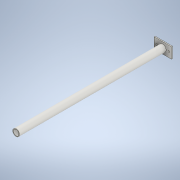
# Autodesk Inventor part: tubo_principal
Saved by Autodesk Inventor 2021 (Build 250183000, 183)
## iProperties
Created: 2022-01-26
Part Number: tubo_principal
Material: Genérico
Document SubType Name: Modeling
Designer: arthu
Density: 1 g/cm^3
Appearance: Acero
Author: arthu
Autodesk Inventor part; units mm, degrees
ref_plane "YZ Plane" through (0, 0, 0) normal (1, 0, 0) x (0, 1, 0)
ref_plane "XZ Plane" through (0, 0, 0) normal (0, 1, 0) x (-1, 0, 0)
ref_plane "XY Plane" through (0, 0, 0) normal (0, 0, 1) x (1, 0, 0)
sketch "Boceto1" plane through (0, 0, 0) normal (0, 0, 1) x (1, 0, 0)
  circle A0 centre (0, 0) radius 25.4
  circle A1 centre (0, 0) radius 20.9
  dimension "d0" = 50.8
  dimension "d1" = 41.8
  constraints: 2 centre point, 2 coincident
  measures "d0" diameter of A0
  measures "d1" diameter of A1
extrude "Extrusión1" add sketch "Boceto1" along normal blind 1095
sketch "Boceto2" plane through (0, 0, 0) normal (0, 0, -1) x (-1, 0, 0)
  line L0 (-65, -40) -> (65, -40)
  line L1 (65, -40) -> (65, 40)
  line L2 (65, 40) -> (-65, 40)
  line L3 (-65, 40) -> (-65, -40)
  line L4 (-65, -40) -> (65, 40) construction
  line L5 (65, -40) -> (-65, 40) construction
  line L6 (-65, 0) -> (-25.4, 0)
  circle A0 centre (0, 0) radius 25.4 projected
  circle A1 centre (-45.2, 0) radius 6.5
  line L7 (25.4, 0) -> (65, 0)
  circle A2 centre (45.2, 0) radius 6.5
  circle A3 centre (0, 0) radius 25.4 projected
  circle A4 centre (0, 0) radius 20.9 projected
  dimension "d4" = 130
  dimension "d5" = 80
  dimension "d6" = 13
  dimension "d7" = 13
  constraints: 16 end point, 6 midpoint, 2 centre point, 2 horizontal, 2 parallel, 2 point on circle, 1 perpendicular
  measures "d4" distance of L2.end L1.end
  measures "d5" distance of L1.end L0.end
  measures "d6" diameter of A1
  measures "d7" diameter of A2
extrude "Extrusión2" add sketch "Boceto2" along normal blind 8 contours L3 L6 A1 A0 L7 A2 L1 L0 | L3 L2 L1 L7 A2 A0 L6 A1 | A0
